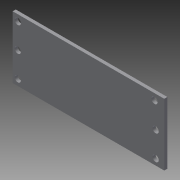
# Autodesk Inventor part: base and top plate real
Saved by Autodesk Inventor 2015 (Build 190159000, 159)
## iProperties
Created: 2015-01-20
Part Number: base and top plate real
Material: Generic
Document SubType Name: Modeling
Designer: mastkee16
Density: 1 g/cm^3
Appearance: Default
Author: mastkee16
Autodesk Inventor part; units mm, degrees
ref_plane "YZ Plane" through (0, 0, 0) normal (1, 0, 0) x (0, 1, 0)
ref_plane "XZ Plane" through (0, 0, 0) normal (0, 1, 0) x (-1, 0, 0)
ref_plane "XY Plane" through (0, 0, 0) normal (0, 0, 1) x (1, 0, 0)
sketch "Sketch1" plane through (0, 0, 0) normal (0, 0, 1) x (1, 0, 0)
  line L0 (-0.2558, -58.1023) -> (154.6842, -58.1023)
  line L1 (154.6842, -58.1023) -> (154.6842, 5.3977)
  line L2 (154.6842, 5.3977) -> (-0.2558, 5.3977)
  line L3 (-0.2558, 5.3977) -> (-0.2558, -58.1023)
  point P0 (0, 0)
  dimension "d0" = 154.94
  dimension "d1" = 63.5
  constraints: 8 end point, 2 parallel, 1 horizontal, 1 perpendicular
  measures "d0" distance of L2.end L1.end
  measures "d1" distance of L2.end L0.start
extrude "Extrusion1" add sketch "Sketch1" along normal blind 3.175
sketch "Sketch2" plane through (0, 0, 3.175) normal (0, 0, 1) x (1, 0, 0)
  line L0 (-0.2558, 5.3977) -> (-0.2558, -58.1023) projected
  line L1 (154.6842, -58.1023) -> (154.6842, 5.3977) projected
  line L2 (154.6842, 5.3977) -> (-0.2558, 5.3977) projected
  point P0 (0, 0)
  point P1 (144.7147, -0.9523)
  point P2 (5.0147, -26.3523)
  point P3 (5.0147, -51.7523)
  point P4 (5.0147, -0.9523)
  point P5 (145.9244, -26.3523)
  point P6 (145.9244, -51.7523)
  dimension "d4" = 139.7
  dimension "d5" = 5.2705
  dimension "d6" = 9.9695
  dimension "d7" = 25.4
  dimension "d8" = 25.4
  dimension "d9" = 25.4
  dimension "d10" = 25.4
  dimension "d11" = 5.2705
  dimension "d12" = 6.35
  dimension "d13" = 63.5
  dimension "d14" = 6.35
  measures "d4" horizontal distance of point (144.715, -0.952) point (5.015, -26.352)
  measures "d5" distance from line of L0 point (5.015, -26.352)
  measures "d6" distance from line of L1 point (144.715, -0.952)
  measures "d7" distance of point (5.015, -26.352) point (5.015, -51.752)
  measures "d8" vertical distance of point (145.924, -26.352) point (144.715, -0.952)
  measures "d9" distance of point (145.924, -51.752) point (145.924, -26.352)
  measures "d10" distance of point (5.015, -26.352) point (5.015, -0.952)
  measures "d11" distance from line of L0 point (5.015, -51.752)
  measures "d12" distance from line of L2 point (144.715, -0.952)
  measures "d13" distance of L0.start L0.end
  measures "d14" distance from line of L2 point (5.015, -0.952)
hole "Hole1" at (144.7147, -0.9523, 3.175) at (5.0147, -26.3523, 3.175) at (5.0147, -51.7523, 3.175) at (5.0147, -0.9523, 3.175) at (145.9244, -26.3523, 3.175) at (145.9244, -51.7523, 3.175) direction (0, 0, -1) diameter 6.35 end through all
body "Solid1"
